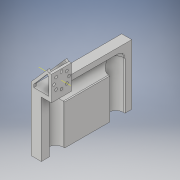
# Autodesk Inventor part: relicmold
Saved by Autodesk Inventor 2017 (Build 210142000, 142)
## iProperties
Created: 2018-02-23
Part Number: relicmold
Material: Generic
Document SubType Name: Modeling
Designer: User
Density: 1 g/cm^3
Appearance: Default
Author: User
Autodesk Inventor part; units mm, degrees
ref_plane "YZ Plane" through (0, 0, 0) normal (1, 0, 0) x (0, 1, 0)
ref_plane "XZ Plane" through (0, 0, 0) normal (0, 1, 0) x (-1, 0, 0)
ref_plane "XY Plane" through (0, 0, 0) normal (0, 0, 1) x (1, 0, 0)
sketch "Sketch1" plane through (0, 0, 0) normal (1, 0, 0) x (0, 1, 0)
  line L0 (0, 0) -> (76.2, 0)
  line L1 (76.2, 0) -> (76.2, -114.3)
  line L2 (76.2, -114.3) -> (0, -114.3)
  line L3 (0, -114.3) -> (0, 0)
  dimension "d0" = 76.2
  dimension "d1" = 114.3
  constraints: 8 end point, 2 parallel, 1 horizontal, 1 perpendicular
  measures "d0" distance of L1.end L2.end
  measures "d1" distance of L0.end L1.end
extrude "Extrusion1" add sketch "Sketch1" along normal blind 12.7
sketch "Sketch2" plane through (12.7, 0, 0) normal (1, 0, 0) x (0, 0, -1)
  line L0 (0, 76.2) -> (0, 0) projected
  line L1 (0, 76.2) -> (25.4, 76.2)
  line L2 (25.4, 76.2) -> (25.4, 70.5404)
  line L3 (25.4, 70.5404) -> (0, 70.5404)
  line L4 (0, 70.5404) -> (0, 76.2)
  dimension "d4" = 25.4
  constraints: 8 end point, 2 parallel, 1 horizontal, 1 perpendicular
  measures "d4" distance of L2.end L3.end
extrude "Extrusion2" add sketch "Sketch2" along normal blind 12.7
sketch "Sketch3" plane through (0, 76.2, 0) normal (0, 1, 0) x (1, 0, 0)
  line L0 (0, 0) -> (0, 114.3) projected
  line L1 (0, 0) -> (25.4, 0) projected
  line L2 (25.4, 25.4) -> (25.4, 0) projected
  line L3 (12.7, 25.4) -> (25.4, 25.4) projected
  line L4 (12.7, 114.3) -> (12.7, 25.4) projected
  line L5 (0, 114.3) -> (12.7, 114.3) projected
  line L6 (12.7, 25.4) -> (25.4, 25.4) projected
  line L7 (22.225, 25.4) -> (22.225, 0)
  line L8 (0, 0) -> (25.4, 0) projected
  dimension "d8" = 3.175
  constraints: 2 end point, 2 point on line, 1 parallel
  measures "d8" distance between parallel lines of L2 L7
extrude "Extrusion3" add sketch "Sketch3" along normal blind 25.4 contours L7 L3 L2 L1
sketch "Sketch4" plane through (0, 0, 0) normal (0, 0, 1) x (1, 0, 0)
  line L0 (0, 76.2) -> (22.225, 76.2) projected
  line L1 (0, 76.2) -> (22.225, 101.6)
  line L2 (22.225, 101.6) -> (19.8356, 103.6908)
  line L3 (19.8356, 103.6908) -> (0, 81.0215)
  line L4 (22.225, 101.6) -> (25.4, 101.6) projected
  line L5 (22.225, 76.2) -> (22.225, 101.6) projected
  line L6 (0, 76.2) -> (0, 81.0215)
  line L7 (22.225, 97.3812) -> (20.1342, 99.2106)
  line L8 (3.175, 76.2) -> (3.175, 79.8286)
  point P0 (0, 0)
  dimension "d11" = 3.175
  dimension "d12" = 3.175
  dimension "d13" = 3.175
  constraints: 12 end point, 6 point on line, 3 perpendicular, 1 parallel, 1 vertical
  measures "d11" distance of L2.end L1.end
  measures "d12" distance from line of L1.end L7
  measures "d13" distance from line of L0.start L8
extrude "Extrusion4" add sketch "Sketch4" against normal blind 3.175 contours L1 L8 L0 | L6 L3 L2 L1 | L1 L5 L7
ref_plane "Work Plane1" through (12.7, 70.5404, -12.7) normal (0, 0, -1) x (-1, 0, 0)
mirror "Mirror1" about plane through (12.7, 70.5404, -12.7) normal (0, 0, -1) of "Extrusion4"
sketch "Sketch5" plane through (25.4, 0, 0) normal (1, 0, 0) x (0, 0, -1)
  line L0 (0, 70.5404) -> (0, 101.6) projected
  line L1 (0, 70.5404) -> (25.4, 70.5404) projected
  line L2 (25.4, 70.5404) -> (25.4, 101.6) projected
  line L3 (0, 101.6) -> (25.4, 101.6) projected
  circle A0 centre (12.7, 88.9) radius 6.35
  line L4 (0, 76.2) -> (25.4, 76.2) projected
  circle A1 centre (12.7, 98.425) radius 1.778
  point P0 (0, 0)
  dimension "d16" = 12.7
  dimension "d17" = 25.4
  dimension "d18" = 25.4
  dimension "d19" = 12.7
  dimension "d20" = 12.7
  dimension "d21" = 3.556
  dimension "d22" = 9.525
  constraints: 2 centre point
  measures "d16" diameter of A0
  measures "d17" distance of L0.start L1.end
  measures "d18" distance between parallel lines of L3 L4
  measures "d19" distance from line of A0.centre L4
  measures "d20" distance from line of L2 A0.centre
  measures "d21" diameter of A1
  measures "d22" distance of A0.centre A1.centre
extrude "Extrusion5" cut sketch "Sketch5" against normal blind 3.175 contours A1
pattern_circular "Circular Pattern1" count 8 over 360 about axis through (25.4, 88.9, -12.7) along (1, 0, 0) of "Extrusion5"
sketch "Sketch6" plane through (0, 0, 0) normal (-1, 0, 0) x (0, 0, 1)
  line L0 (0, 0) -> (-114.3, 0) projected
  line L1 (-20.0153, 0) -> (-20.0153, 59.8716) construction
  line L2 (-10.4903, 0) -> (-10.4903, 59.8716)
  line L3 (-29.5403, 59.8716) -> (-29.5403, 0)
  arc A0 (-29.5403, 0) -> (-10.4903, 0) centre (-20.0153, 0) ccw
  arc A1 (-10.4903, 59.8716) -> (-29.5403, 59.8716) centre (-20.0153, 59.8716) ccw
  line L4 (-20.0153, 59.8716) -> (-96.2153, 59.8716) construction
  line L5 (-20.0153, 69.3966) -> (-96.2153, 69.3966)
  line L6 (-96.2153, 50.3466) -> (-20.0153, 50.3466)
  arc A2 (-20.0153, 50.3466) -> (-20.0153, 69.3966) centre (-20.0153, 59.8716) ccw
  arc A3 (-96.2153, 69.3966) -> (-96.2153, 50.3466) centre (-96.2153, 59.8716) ccw
  line L7 (-96.2153, 59.8716) -> (-96.2153, 0) construction
  line L8 (-105.7403, 59.8716) -> (-105.7403, 0)
  line L9 (-86.6903, 0) -> (-86.6903, 59.8716)
  arc A4 (-86.6903, 59.8716) -> (-105.7403, 59.8716) centre (-96.2153, 59.8716) ccw
  arc A5 (-105.7403, 0) -> (-86.6903, 0) centre (-96.2153, 0) ccw
  line L10 (-114.3, 0) -> (-114.3, 76.2) projected
  line L11 (0, 0) -> (0, 81.0215) projected
  point P0 (-20.0153, 29.9358)
  point P1 (-58.1153, 59.8716)
  point P2 (-96.2153, 29.9358)
  dimension "d28" = 19.05
  dimension "d29" = 76.2
  dimension "d30" = 19.05
  dimension "d31" = 19.05
  dimension "d32" = 95.25
  dimension "d36" = 116.2307
  dimension "d37" = 10.4903
  constraints: 24 end point, 12 point on circle, 12 tangent, 6 centre point, 3 midpoint, 3 parallel, 3 perpendicular, 2 point on line
  measures "d28" diameter of A1
  measures "d29" distance of L1.end L4.end
  measures "d30" diameter of A3
  measures "d31" diameter of A5
  measures "d32" distance between parallel lines of L2 L8
  measures "d37" distance between parallel lines of L11 L2
sketch "Sketch7" plane through (12.7, 0, 0) normal (1, 0, 0) x (0, 0, -1)
  line L0 (25.4, 70.5404) -> (0, 70.5404) projected
  line L1 (0, 70.5404) -> (0, 0) projected
  line L2 (0, 0) -> (114.3, 0) construction
  line L3 (114.3, 0) -> (114.3, 76.2) projected
  line L4 (114.3, 76.2) -> (25.4, 76.2) projected
  line L5 (25.4, 76.2) -> (25.4, 70.5404) projected
  line L6 (105.7403, 59.8716) -> (105.7403, 0) projected
  line L7 (20.0153, 69.3966) -> (96.2153, 69.3966) projected
  line L8 (0, 0) -> (0, 81.0215) projected
  line L9 (0, 81.0215) -> (3.175, 81.0215) projected
  line L10 (3.175, 76.2) -> (3.175, 81.0215) projected
  line L11 (3.175, 76.2) -> (22.225, 76.2) projected
  line L12 (22.225, 76.2) -> (22.225, 81.0215) projected
  line L13 (25.4, 81.0215) -> (22.225, 81.0215) projected
  line L14 (25.4, 81.0215) -> (25.4, 76.2) projected
  line L15 (25.4, 76.2) -> (114.3, 76.2) projected
  line L16 (114.3, 76.2) -> (114.3, 0) projected
  line L17 (114.3, 0) -> (0, 0) projected
  arc A0 (105.7403, 59.8716) -> (86.6903, 59.8716) centre (96.2153, 59.8716) ccw projected
  arc A1 (96.2153, 50.3466) -> (96.2153, 69.3966) centre (96.2153, 59.8716) ccw projected
  line L18 (96.2153, 50.3466) -> (20.0153, 50.3466) projected
  line L19 (86.6903, 0) -> (86.6903, 59.8716) projected
  arc A2 (86.6903, 0) -> (105.7403, 0) centre (96.2153, 0) ccw projected
  arc A3 (10.4903, 0) -> (29.5403, 0) centre (20.0153, 0) ccw projected
  line L20 (29.5403, 59.8716) -> (29.5403, 0) projected
  line L21 (10.4903, 0) -> (10.4903, 59.8716) projected
  arc A4 (29.5403, 59.8716) -> (10.4903, 59.8716) centre (20.0153, 59.8716) ccw projected
  arc A5 (20.0153, 69.3966) -> (20.0153, 50.3466) centre (20.0153, 59.8716) ccw projected
extrude "Extrusion7" cut sketch "Sketch7" against normal blind 11.43 contours L21 A5 L18 L20 L17 | L17 A3 | A4 L20 L18 A5 | L17 L19 L18 A1 L6 | A2 L17 | L20 A4 L7 A0 L19 L18 | A1 L18 L19 A0
fillet "Fillet2" radius 9.525 8 edges at (1.27, 66.6068, -102.9505) (1.27, 29.9358, -105.7403) (1.27, 66.6068, -13.2801) (1.27, 29.9358, -10.4903) (1.27, 69.3966, -58.1153) (1.27, 25.1733, -86.6903) (1.27, 50.3466, -58.1153) (1.27, 25.1733, -29.5403)
equation "\"d12\" = d13"
equation "\"d19\" = 0.5 * d18"
equation "\"d20\" = 0.5 * d17"
equation "\"d28\" = d31"
equation "\"d30\" = d31"
equation "\"d37\" = -0.5 * d32 + 0.5 * d36"
body "Solid1"
